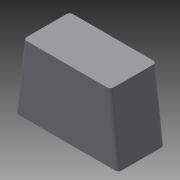
# Autodesk Inventor part: Box MKIV Version 1
Saved by Autodesk Inventor 2013 (Build 170138000, 138)
## iProperties
Created: 2014-12-24
Part Number: Box MKIV Version 1
Material: Generic
Document SubType Name: Modeling
Designer: Zep
Density: 1 g/cm^3
Author: Zep
Autodesk Inventor part; units mm, degrees
ref_plane "YZ Plane" through (0, 0, 0) normal (1, 0, 0) x (0, 1, 0)
ref_plane "XZ Plane" through (0, 0, 0) normal (0, 1, 0) x (-1, 0, 0)
ref_plane "XY Plane" through (0, 0, 0) normal (0, 0, 1) x (1, 0, 0)
sketch "Sketch1" plane through (0, 0, 0) normal (0, 0, 1) x (1, 0, 0)
  line L0 (0, 0) -> (129, 0)
  line L1 (129, 0) -> (129, 85)
  line L2 (129, 85) -> (0, 85)
  line L3 (0, 85) -> (0, 0)
  line L4 (0, 85) -> (10, 85)
  line L5 (10, 85) -> (0, 0)
  line L6 (129, 85) -> (119, 85)
  line L7 (119, 85) -> (129, 0)
  dimension "d0" = 129
  dimension "d1" = 85
  dimension "d2" = 10
  dimension "d3" = 10
  constraints: 16 end point, 2 parallel, 2 point on line, 1 horizontal, 1 perpendicular
  measures "d0" distance of L2.end L1.end
  measures "d1" distance of L1.end L0.end
  measures "d2" distance of L2.end L4.end
  measures "d3" distance of L1.end L6.end
extrude "Extrusion1" add sketch "Sketch1" against normal blind 58 contours L5 L2 L7 L0
fillet "Fillet1" radius 4 4 edges at (5, 42.5, 0) (124, 42.5, 0) (124, 42.5, -58) (5, 42.5, -58)
shell "Shell1" thickness 3 removed faces 1 at (44.3425, 0, -19.3333)
sketch "Sketch2" plane through (0, 0, -58) normal (0, 0, -1) x (-1, 0, 0)
  line L0 (-14.0276, 85) -> (-114.9724, 85) projected
  line L1 (-124.9724, 0) -> (-4.0276, 0) projected
  line L2 (-22.0276, 0) -> (-22.0276, 55)
  line L3 (-22.0276, 55) -> (-22.0276, 55)
  circle A0 centre (-22.0276, 55) radius 7.829
  line L4 (-29.8566, 55) -> (-36.5566, 55)
  line L5 (-36.5566, 55) -> (-44.4066, 55)
  circle A1 centre (-44.4066, 55) radius 7.85
  line L6 (-52.2566, 55) -> (-87.7566, 55)
  circle A2 centre (-87.7566, 55) radius 22.5
  line L7 (-4.0276, 0) -> (-22.0276, 0)
  point P0 (0, 0)
  dimension "d10" = 15.6579
  dimension "d8" = 55
  dimension "d9" = 0
  dimension "d11" = 6.7
  dimension "d12" = 7.85
  dimension "d13" = 35.5
  dimension "d14" = 45
  dimension "d15" = 18
  constraints: 12 end point, 3 coincident, 3 collinear, 2 centre point, 2 perpendicular, 2 point on circle, 2 point on line, 1 horizontal alignment, 2 other
  measures "d8" distance of L2.start L2.end
  measures "d9" distance of L2.end L3.end
  measures "d11" distance of L4.start L4.end
  measures "d12" distance of L4.end L5.end
  measures "d13" distance of L6.start L6.end
  measures "d14" diameter of A2
  measures "d15" distance of L1.end L2.start
extrude "Extrusion2" cut sketch "Sketch2" against normal blind 5
chamfer "Chamfer1" distance 3 distance2 1 1 edges at (110.2566, 55, -58) measured on face at (69.5927, 11.3207, -58)
body "Solid1"
